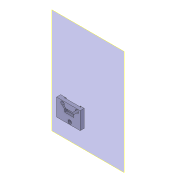
# Autodesk Inventor part: cellSTORM_v5_chiptray_new_0_22.4
Saved by Autodesk Inventor 2019.4 (Build 234330000, 330)
## iProperties
Created: 2020-05-10
Part Number: cellSTORM_v5_chiptray_new_0_22.4
Material: Generic
Document SubType Name: Modeling
Designer: diederichbenedict
Density: 1 g/cm^3
Appearance: Default
Author: diederichbenedict
Autodesk Inventor part; units mm, degrees
ref_plane "YZ Plane" through (0, 0, 0) normal (1, 0, 0) x (0, 1, 0)
ref_plane "XZ Plane" through (0, 0, 0) normal (0, 1, 0) x (-1, 0, 0)
ref_plane "XY Plane" through (0, 0, 0) normal (0, 0, 1) x (1, 0, 0)
ref_plane "Work Plane1" through (52.5141, 202.7033, 6.4479) normal (0, 0, -1) x (0, 1, 0)
sketch "Sketch1" plane through (52.5141, 202.7033, 6.4479) normal (0, 0, -1) x (0, 1, 0)
  circle A0 centre (-59.8114, -30.5) radius 1.4 construction
  circle A1 centre (-38.8114, -18.3756) radius 1.4 projected
  circle A2 centre (-38.8114, -42.6244) radius 1.4 construction
  circle A3 centre (41, 0) radius 1.65 projected
  circle A4 centre (-9, 0) radius 1.65 projected
  circle A5 centre (-9, 50) radius 1.65 projected
  circle A6 centre (41, 50) radius 1.65 projected
  circle A7 centre (16, 50) radius 1.65 projected
  circle A8 centre (-9, 25) radius 1.65 projected
  circle A9 centre (16, 0) radius 1.65 projected
  circle A10 centre (41, 25) radius 1.65 projected
  line L0 (80, 55) -> (-80, 55) projected
  line L1 (-80, 55) -> (-80, -55) projected
  line L2 (-80, -55) -> (80, -55) projected
  line L3 (80, -55) -> (80, 55) projected
  line L4 (-36.5, 0) -> (-36.5, -50) projected
  line L5 (-14, 0) -> (-36.5, 0) projected
  line L6 (-14, -5) -> (-14, 0) projected
  line L7 (72, -5) -> (-14, -5) projected
  line L8 (72, -50) -> (72, -5) projected
  line L9 (-36.5, -50) -> (72, -50) projected
  line L10 (-4, 45) -> (-4, 5) projected
  line L11 (36, 45) -> (-4, 45) projected
  line L12 (36, 5) -> (36, 45) projected
  line L13 (-4, 5) -> (36, 5) projected
  line L14 (-64.5989, -17.0433) -> (-64.5989, -57.0433) construction
  line L15 (-64.5989, -57.0433) -> (-34.5989, -57.0433) construction
  line L16 (-34.5989, -57.0433) -> (-34.5989, -17.0433) construction
  line L17 (-34.5989, -17.0433) -> (-64.5989, -17.0433) construction
  line L18 (-34.8114, -13.0433) -> (-63.8114, -13.0433)
  line L19 (-63.8114, -13.0433) -> (-63.8114, -52.6244)
  line L20 (-63.8114, -52.6244) -> (-34.8114, -52.6244)
  line L21 (-34.8114, -52.6244) -> (-34.8114, -13.0433)
  circle A11 centre (-59.8114, -30.5) radius 2.95
  circle A12 centre (-38.8114, -18.3756) radius 2.95
  circle A13 centre (-38.8114, -42.6244) radius 2.95 construction
  line L22 (-36.5, -35.1157) -> (-41.75, -35.1157) construction
  line L23 (-41.75, -35.1157) -> (-41.75, -38.5657) construction
  line L24 (-41.75, -38.5657) -> (-56.86, -38.5657) construction
  line L25 (-56.86, -38.5657) -> (-56.86, -35.1157) construction
  line L26 (-56.86, -35.1157) -> (-60.26, -35.1157) construction
  line L27 (-60.26, -35.1157) -> (-60.26, -52.0657) construction
  line L28 (-60.26, -52.0657) -> (-36.5, -52.0657) construction
  line L29 (-36.5, -52.0657) -> (-36.5, -35.1157) construction
  line L30 (-41.75, -28.3657) -> (-36.5, -28.3657) construction
  line L31 (-36.5, -28.3657) -> (-36.5, -25.0657) construction
  line L32 (-36.5, -25.0657) -> (-60.26, -25.0657) construction
  line L33 (-60.26, -25.0657) -> (-60.26, -28.3657) construction
  line L34 (-60.26, -28.3657) -> (-56.86, -28.3657) construction
  line L35 (-56.86, -28.3657) -> (-56.86, -27.0942) construction
  line L36 (-56.86, -27.0942) -> (-41.75, -27.0942) construction
  line L37 (-41.75, -27.0942) -> (-41.75, -28.3657) construction
  line L38 (-56.86, -35.1157) -> (-60.26, -35.1157) construction
  line L39 (-56.86, -38.5657) -> (-56.86, -35.1157) construction
  line L40 (-41.75, -38.5657) -> (-56.86, -38.5657) construction
  line L41 (-41.75, -35.1157) -> (-41.75, -38.5657) construction
  line L42 (-36.5, -35.1157) -> (-41.75, -35.1157) construction
  line L43 (-36.5, -35.05) -> (-36.5, -35.1157) construction
  line L44 (-36.5, -35.05) -> (-56.86, -35.05) construction
  line L45 (-36.5, -34.78) -> (-36.5, -35.05) construction
  line L46 (-36.5, -34.78) -> (-56.86, -34.78) construction
  line L47 (-36.5, -34.51) -> (-36.5, -34.78) construction
  line L48 (-36.5, -34.51) -> (-56.86, -34.51) construction
  line L49 (-36.5, -34.24) -> (-36.5, -34.51) construction
  line L50 (-36.5, -34.24) -> (-56.86, -34.24) construction
  line L51 (-36.5, -33.97) -> (-36.5, -34.24) construction
  line L52 (-36.5, -33.97) -> (-56.86, -33.97) construction
  line L53 (-36.5, -33.7) -> (-36.5, -33.97) construction
  line L54 (-36.5, -33.7) -> (-56.86, -33.7) construction
  line L55 (-36.5, -33.43) -> (-36.5, -33.7) construction
  line L56 (-36.5, -33.43) -> (-56.86, -33.43) construction
  line L57 (-36.5, -33.16) -> (-36.5, -33.43) construction
  line L58 (-36.5, -33.16) -> (-56.86, -33.16) construction
  line L59 (-36.5, -32.89) -> (-36.5, -33.16) construction
  line L60 (-36.5, -32.89) -> (-56.86, -32.89) construction
  line L61 (-36.5, -32.62) -> (-36.5, -32.89) construction
  line L62 (-36.5, -32.62) -> (-56.86, -32.62) construction
  line L63 (-36.5, -32.35) -> (-36.5, -32.62) construction
  line L64 (-36.5, -32.35) -> (-56.86, -32.35) construction
  line L65 (-36.5, -32.08) -> (-36.5, -32.35) construction
  line L66 (-36.5, -32.08) -> (-56.86, -32.08) construction
  line L67 (-36.5, -31.81) -> (-36.5, -32.08) construction
  line L68 (-36.5, -31.81) -> (-56.86, -31.81) construction
  line L69 (-36.5, -31.54) -> (-36.5, -31.81) construction
  line L70 (-36.5, -31.54) -> (-56.86, -31.54) construction
  line L71 (-36.5, -31.27) -> (-36.5, -31.54) construction
  line L72 (-36.5, -31.27) -> (-56.86, -31.27) construction
  line L73 (-36.5, -31) -> (-36.5, -31.27) construction
  line L74 (-36.5, -31) -> (-56.86, -31) construction
  line L75 (-36.5, -30.73) -> (-36.5, -31) construction
  line L76 (-36.5, -30.73) -> (-56.86, -30.73) construction
  line L77 (-36.5, -30.46) -> (-36.5, -30.73) construction
  line L78 (-36.5, -30.46) -> (-56.86, -30.46) construction
  line L79 (-36.5, -30.19) -> (-36.5, -30.46) construction
  line L80 (-36.5, -30.19) -> (-56.86, -30.19) construction
  line L81 (-36.5, -29.92) -> (-36.5, -30.19) construction
  line L82 (-36.5, -29.92) -> (-56.86, -29.92) construction
  line L83 (-36.5, -29.65) -> (-36.5, -29.92) construction
  line L84 (-36.5, -29.65) -> (-56.86, -29.65) construction
  line L85 (-36.5, -29.38) -> (-36.5, -29.65) construction
  line L86 (-36.5, -29.38) -> (-56.86, -29.38) construction
  line L87 (-36.5, -29.11) -> (-36.5, -29.38) construction
  line L88 (-36.5, -29.11) -> (-56.86, -29.11) construction
  line L89 (-36.5, -28.84) -> (-36.5, -29.11) construction
  line L90 (-36.5, -28.84) -> (-56.86, -28.84) construction
  line L91 (-36.5, -28.3657) -> (-36.5, -28.84) construction
  line L92 (-41.75, -28.3657) -> (-36.5, -28.3657) construction
  line L93 (-41.75, -27.0942) -> (-41.75, -28.3657) construction
  line L94 (-56.86, -27.0942) -> (-41.75, -27.0942) construction
  line L95 (-56.86, -28.3657) -> (-56.86, -27.0942) construction
  line L96 (-60.26, -28.3657) -> (-56.86, -28.3657) construction
  line L97 (-60.26, -35.1157) -> (-60.26, -28.3657) construction
  line L98 (-60.26, -25.0657) -> (-36.5, -25.0657) construction
  line L99 (-36.5, -25.0657) -> (-36.5, -52.0657) construction
  line L100 (-60.26, -52.0657) -> (-60.26, -25.0657) construction
  line L101 (-57.1632, -22.5233) -> (-33.4032, -22.5233) construction
  line L102 (-33.4032, -22.5233) -> (-33.4032, -49.5233) construction
  line L103 (-33.4032, -49.5233) -> (-57.1632, -49.5233) construction
  line L104 (-57.1632, -49.5233) -> (-57.1632, -22.5233) construction
  circle A14 centre (-38.8114, -42.6244) radius 2.95
  point P0 (-202.7033, -52.5141)
  point P1 (-56.7146, -27.9576)
  dimension "d0" = 4
  dimension "d2" = 4
  dimension "d3" = 4
  dimension "d4" = 5.9
  dimension "d5" = 5.9
  dimension "d6" = 5.9
  dimension "d10" = 10
  constraints: 22 end point, 5 parallel, 4 centre point, 4 coincident, 3 horizontal, 3 perpendicular, 1 concentric, 1 other
  measures "d0" distance between parallel lines of L18 L17
  measures "d2" distance from line of L21 A1.centre
  measures "d3" distance from line of L19 A0.centre
  measures "d4" diameter of A11
  measures "d5" diameter of A12
  measures "d6" diameter of A13
  measures "d10" distance from line of L20 A2.centre
extrude "Extrusion1" add sketch "Sketch1" along normal blind 4 contours L18 L21 L9 L4 A14 A12 | L4 A12 A14 L9 L21 L20 L19 L18
sketch "Sketch2" plane through (52.5141, 202.7033, 2.4479) normal (0, 0, -1) x (-1, 0, 0)
  circle A0 centre (42.6244, -38.8114) radius 2.95 projected
  circle A1 centre (18.3756, -38.8114) radius 2.95 projected
  circle A2 centre (30.5, -59.8114) radius 2.95 projected
  line L0 (13.0433, -34.8114) -> (13.0433, -63.8114) projected
  line L1 (13.0433, -63.8114) -> (52.6244, -63.8114) projected
  line L2 (52.6244, -63.8114) -> (52.6244, -34.8114) projected
  line L3 (52.6244, -34.8114) -> (13.0433, -34.8114) projected
  point P0 (52.5141, -202.7033)
extrude "Extrusion2" add sketch "Sketch2" along normal blind 1.5 contours A0 | A1 | A2 | L3 L2 L1 L0
sketch "Sketch3" plane through (-0.1103, 138.8919, 6.4479) normal (0, -1, 0) x (1, 0, 0)
  line L0 (39.581, 0) -> (0, 0) projected
  line L1 (0, 0) -> (0, -5.5) projected
  line L2 (39.581, -5.5) -> (0, -5.5) projected
  line L3 (39.581, 0) -> (39.581, -5.5) projected
  line L4 (17.5087, -7.4479) -> (17.5087, -6.8479) construction
  line L5 (17.5087, -6.8479) -> (24.2587, -6.8479) construction
  line L6 (24.2587, -6.8479) -> (24.2587, -7.4479) construction
  line L7 (27.5587, -7.4479) -> (24.2587, -7.4479) construction
  line L8 (27.5587, -6.4479) -> (27.5587, -7.4479) construction
  line L9 (27.5587, -6.4479) -> (0.5587, -6.4479) construction
  line L10 (0.5587, -6.4479) -> (0.5587, -7.4479) construction
  line L11 (17.5087, -7.4479) -> (0.5587, -7.4479) construction
  line L12 (39.581, 0) -> (39.581, -5.5) projected
  line L13 (39.581, -5.5) -> (34.8694, -5.5)
  line L14 (34.8694, -5.5) -> (34.8694, -6)
  line L15 (34.8694, -6.8) -> (39.581, -6.8)
  line L16 (39.581, -6.8) -> (39.581, -5.5)
  line L17 (39.581, -6.8) -> (32.6714, -6.8)
  line L18 (32.6714, -6.8) -> (34.8694, -6)
  line L19 (12.6726, -5.5) -> (12.6726, -6.5) projected
  line L20 (0, 0) -> (0, -5.5) projected
  line L21 (0, -5.5) -> (8.1109, -5.5)
  line L22 (8.1109, -6.8) -> (0, -6.8)
  line L23 (0, -6.8) -> (0, -5.5)
  line L24 (9.7957, -6.8) -> (8.1109, -6.8)
  line L25 (0, -5.5) -> (39.581, -5.5) projected
  line L26 (9.7957, -6.8) -> (7.5977, -6)
  line L27 (7.5977, -6) -> (7.5977, -5.5)
  line L28 (8.8957, -5.5) -> (33.4957, -5.5) construction
  line L29 (33.4957, -5.5) -> (33.4957, -6.5) construction
  line L30 (33.4957, -6.5) -> (8.8957, -6.5) construction
  line L31 (8.8957, -6.5) -> (8.8957, -5.5) construction
  point P0 (8.981, -5.5)
  dimension "d42" = 1.3
  dimension "d43" = 110
  dimension "d45" = 0.5
  dimension "d46" = 0.5
  dimension "d47" = 110
  dimension "d48" = 24.6
  dimension "d49" = 1
  dimension "d50" = 0.9
  dimension "d51" = 0
  constraints: 32 end point, 6 parallel, 4 horizontal, 3 point on line, 2 perpendicular, 1 collinear, 1 vertical
  measures "d42" distance between parallel lines of L25 L22
  measures "d43" angle of L14 L18
  measures "d45" distance from line of L14.end L25
  measures "d46" distance from line of L2 L26.end
  measures "d47" angle of L27 L26
  measures "d48" distance of L29.end L30.end
  measures "d49" distance of L28.end L29.end
  measures "d50" distance from line of L24.start L31
  measures "d51" distance between parallel lines of L22 L15
extrude "Extrusion3" add sketch "Sketch3" against normal up to surface (29 mm away) contours L16 L15 L17 L18 L14 L2 | L2 L27 L26 L24 L22 L23
sketch "Sketch6" plane through (52.5141, 202.7033, 6.4479) normal (0, 0, 1) x (1, 0, 0)
  line L0 (-13.0433, -34.8114) -> (-13.0433, -63.8114) projected
  line L1 (-52.6244, -34.8114) -> (-13.0433, -34.8114) projected
  line L2 (-52.6244, -63.8114) -> (-52.6244, -34.8114) projected
  line L3 (-13.0433, -63.8114) -> (-52.6244, -63.8114) projected
  line L4 (-23.5962, -45.8071) -> (-17.5454, -39.7563)
  line L5 (-17.5454, -39.7563) -> (-19.6668, -37.635)
  line L6 (-19.6668, -37.635) -> (-25.7175, -43.6858)
  line L7 (-25.7175, -43.6858) -> (-23.5962, -45.8071)
  line L8 (-23.5962, -45.8071) -> (-19.6668, -37.635) construction
  line L9 (-17.5454, -39.7563) -> (-25.7175, -43.6858) construction
  line L10 (-39.0797, -45.8071) -> (-43.9064, -40.9803)
  line L11 (-43.9064, -40.9803) -> (-41.7851, -38.859)
  line L12 (-41.7851, -38.859) -> (-36.9583, -43.6858)
  line L13 (-36.9583, -43.6858) -> (-39.0797, -45.8071)
  line L14 (-39.0797, -45.8071) -> (-41.7851, -38.859) construction
  line L15 (-43.9064, -40.9803) -> (-36.9583, -43.6858) construction
  line L16 (-25.7175, -43.6858) -> (-36.9583, -43.6858)
  line L17 (-23.5962, -45.8071) -> (-23.5962, -49.9899)
  line L18 (-23.5962, -49.9899) -> (-39.0797, -49.9899)
  line L19 (-39.0797, -49.9899) -> (-39.0797, -45.8071)
  point P0 (-52.5141, -202.7033)
  point P1 (-21.6315, -41.7211)
  point P2 (-40.4324, -42.333)
  dimension "d35" = 3
  dimension "d36" = 3
  dimension "d37" = 45
  dimension "d38" = 0
  constraints: 32 end point, 5 parallel, 4 midpoint, 4 perpendicular, 1 vertical
  measures "d35" distance of L5.end L4.end
  measures "d36" distance of L10.end L11.end
  measures "d37" angle of L1 L12
  measures "d38" vertical distance of L12.end L6.end
extrude "Extrusion6" cut sketch "Sketch6" against normal up to surface (4 mm away) contours L7 L6 L5 L4 | L17 L18 L19 L13 L16 L7 | L13 L10 L11 L12
body "Solid1"
